Autodesk Fusion 360 part; units mm, degrees
(part 4 of 5)
sketch "Content (4)" plane through (0, 0, 0) normal (0, 0, 1) x (1, 0, 0) in component "Back"
  line L0 (128, -33) -> (128, -39)
  line L1 (116, -39) -> (116, -33)
  circle A0 centre (172, -18) radius 1.75
  circle A1 centre (182, -28) radius 1.75
  circle A2 centre (182, -18) radius 1.75
  line L2 (2, -6) -> (2, -66) construction
  line L3 (119, -30) -> (125, -30)
  line L4 (242, -6) -> (2, -6) construction
  line L5 (2, -66) -> (242, -66) construction
  circle A3 centre (56, -27) radius 1.5
  circle A4 centre (172, -28) radius 1.75
  circle A5 centre (71, -17) radius 1.5
  circle A6 centre (56, -17) radius 1.5
  circle A7 centre (46, -32) radius 1.5
  circle A8 centre (223.2, -48) radius 5.5
  line L6 (242, -66) -> (242, -6) construction
  circle A9 centre (66, -32) radius 1.5
  circle A10 centre (66, -22) radius 1.5
  circle A11 centre (61, -32) radius 1.5
  circle A12 centre (41, -27) radius 1.5
  circle A13 centre (71, -32) radius 1.5
  circle A14 centre (46, -17) radius 1.5
  circle A15 centre (56, -22) radius 1.5
  circle A16 centre (66, -17) radius 1.5
  circle A17 centre (56, -32) radius 1.5
  circle A18 centre (66, -27) radius 1.5
  circle A19 centre (61, -22) radius 1.5
  circle A20 centre (61, -17) radius 1.5
  circle A21 centre (46, -22) radius 1.5
  circle A22 centre (51, -22) radius 1.5
  line L7 (125, -42) -> (119, -42)
  circle A23 centre (41, -32) radius 1.5
  circle A24 centre (51, -32) radius 1.5
  circle A25 centre (41, -17) radius 1.5
  circle A26 centre (71, -27) radius 1.5
  circle A27 centre (46, -27) radius 1.5
  circle A28 centre (51, -27) radius 1.5
  circle A29 centre (61, -27) radius 1.5
  circle A30 centre (51, -17) radius 1.5
  circle A31 centre (41, -22) radius 1.5
  circle A32 centre (71, -22) radius 1.5
  line L8 (0, 1.75) -> (0, 22.5) construction
  line L9 (1.75, 0) -> (22.5, 0) construction
  circle A33 centre (192, -18) radius 1.75
  circle A34 centre (202, -18) radius 1.75
  circle A35 centre (192, -28) radius 1.75
  circle A36 centre (202, -28) radius 1.75
  line L10 (14.1495, -52.3784) -> (48.441, -52.3784) construction
  line L11 (48.441, -52.3784) -> (48.441, -46.5889) construction
  line L12 (48.441, -46.5889) -> (14.1495, -46.5889) construction
  line L13 (14.1495, -46.5889) -> (14.1495, -52.3784) construction
  arc A37 (119, -30) -> (116, -33) centre (119, -33) ccw
  arc A38 (128, -33) -> (125, -30) centre (125, -33) ccw
  arc A39 (125, -42) -> (128, -39) centre (125, -39) ccw
  arc A40 (116, -39) -> (119, -42) centre (119, -39) ccw
  line L14 (227, -16) -> (227, -26)
  line L15 (220.6, -14) -> (225, -14)
  line L16 (225, -28) -> (220.6, -28)
  line L17 (218.6, -26) -> (218.6, -16)
  arc A41 (220.6, -14) -> (218.6, -16) centre (220.6, -16) ccw
  arc A42 (227, -16) -> (225, -14) centre (225, -16) ccw
  arc A43 (218.6, -26) -> (220.6, -28) centre (220.6, -26) ccw
  arc A44 (225, -28) -> (227, -26) centre (225, -26) ccw
  point P0 (242, -36)
  point P1 (116, -42)
  point P2 (116, -30)
  point P3 (128, -30)
  point P4 (218.6, -28)
  point P5 (218.6, -14)
  point P6 (227, -14)
  point P7 (223.2, -28)
  dimension "d1005" = 5
  dimension "d1006" = 5
  dimension "d1009" = 10
  dimension "d1010" = -10
  dimension "d502" = 240
  dimension "d503" = 60
  dimension "d696" = 18
  dimension "d866" = 12
  dimension "d867" = 12
  dimension "d869" = 24
  dimension "d870" = 3
  dimension "d1039" = 34
  dimension "d1041" = 12
  dimension "d1179" = 18.8
  dimension "d1180" = 114
  dimension "d1183" = 39
  dimension "d1047" = 2
  dimension "d1048" = 6
  dimension "d1561" = 3.5
  dimension "d1562" = 11
  dimension "d1563" = 70
  dimension "d1596" = 3
  dimension "d1597" = 3
  dimension "d1598" = 3
  dimension "d1599" = 3
  dimension "d1646" = 8.4
  dimension "d1647" = 14
  dimension "d1648" = 8
  dimension "d1654" = 2
  dimension "d1655" = 2
  dimension "d1656" = 2
  dimension "d1657" = 2
  dimension "d1658" = 15
  constraint horizontal L5
  constraint vertical L6
  constraint vertical L2
  constraint midpoint P0 L6
  constraint horizontal L4
  constraint horizontal L3
  constraint vertical L0
  constraint horizontal L7
  constraint vertical L1
  constraint coincident P2 L1
  constraint coincident P2 L3
  constraint tangent L1 A37
  constraint tangent L3 A37
  constraint coincident P3 L3
  constraint coincident P3 L0
  constraint tangent L3 A38
  constraint tangent L0 A38
  constraint tangent L0 A39
  constraint tangent L7 A39
  constraint coincident P1 L1
  constraint coincident P1 L7
  constraint tangent L1 A40
  constraint tangent L7 A40
  constraint horizontal L15
  constraint vertical L14
  constraint horizontal L16
  constraint vertical L17
  constraint vertical A8.centre P7
  constraint coincident P5 L17
  constraint coincident P5 L15
  constraint tangent L17 A41
  constraint tangent L15 A41
  constraint coincident P6 L15
  constraint coincident P6 L14
  constraint tangent L15 A42
  constraint tangent L14 A42
  constraint coincident L16 P7
  constraint coincident P4 L17
  constraint coincident P4 L16
  constraint tangent L17 A43
  constraint tangent L16 A43
  constraint tangent L14 A44
  constraint tangent L16 A44
  measures "d502" distance of L5.end L2.end
  measures "d503" distance of L2.end L2.start
  measures "d696" distance of A8.centre L5
  measures "d866" distance of P2 P3
  measures "d867" distance of P1 P2
  measures "d869" distance of L5 L7
  measures "d870" diameter of A23
  measures "d1039" distance of A23.centre L5
  measures "d1041" distance of A0.centre L4
  measures "d1179" distance of A8.centre L6
  measures "d1180" distance of L0 L6
  measures "d1183" distance of A23.centre L2
  measures "d1047" distance of L2 L8
  measures "d1048" distance of L4 L9
  measures "d1561" diameter of A0
  measures "d1562" diameter of A8
  measures "d1563" distance of A0.centre L6
  measures "d1596" radius of A37
  measures "d1597" radius of A38
  measures "d1598" radius of A39
  measures "d1599" radius of A40
  measures "d1646" distance of P5 P6
  measures "d1647" distance of P4 P5
  measures "d1648" distance of L4 L15
  measures "d1654" radius of A41
  measures "d1655" radius of A42
  measures "d1656" radius of A43
  measures "d1657" radius of A44
  measures "d1658" distance of L6 L14
sketch "Content (5)" plane through (0, 0, 0) normal (0, 0, 1) x (1, 0, 0) in component "Right"
  line L0 (-302, 182) -> (-242, 182) construction
  circle A0 centre (-275, 112) radius 5.75
  circle A1 centre (-277, 80) radius 1.75
  circle A2 centre (-287, 100) radius 1.75
  circle A3 centre (-277, 90) radius 1.75
  line L1 (-264.7, 57.5) -> (-267, 57.5)
  line L2 (-267, 45) -> (-264.7, 45)
  circle A4 centre (-287, 90) radius 1.75
  circle A5 centre (-287, 80) radius 1.75
  line L3 (-269, 55.5) -> (-269, 47)
  line L4 (-262.7, 47) -> (-262.7, 55.5)
  circle A6 centre (-297, 151) radius 1
  circle A7 centre (-277, 100) radius 1.75
  circle A8 centre (-297, 61) radius 1
  circle A9 centre (-297, 121) radius 1
  circle A10 centre (-297, 91) radius 1
  line L5 (-242, 182) -> (-242, 0) construction
  circle A11 centre (-297, 31) radius 1
  line L6 (-302, 0) -> (-302, 182) construction
  circle A12 centre (-267, 80) radius 1.75
  line L7 (-242, 0) -> (-302, 0) construction
  circle A13 centre (-267, 90) radius 1.75
  circle A14 centre (-267, 100) radius 1.75
  line L8 (1.75, 0) -> (22.5, 0) construction
  line L9 (0, 1.75) -> (0, 22.5) construction
  arc A15 (-262.7, 55.5) -> (-264.7, 57.5) centre (-264.7, 55.5) ccw
  arc A16 (-267, 57.5) -> (-269, 55.5) centre (-267, 55.5) ccw
  arc A17 (-269, 47) -> (-267, 45) centre (-267, 47) ccw
  arc A18 (-264.7, 45) -> (-262.7, 47) centre (-264.7, 47) ccw
  point P0 (-242, 91)
  point P1 (-262.7, 45)
  point P2 (-272, 0)
  point P3 (-269, 45)
  point P4 (-269, 57.5)
  point P5 (-302, 182)
  point P6 (-272, 182)
  dimension "d960" = -10
  dimension "d961" = -10
  dimension "d964" = 0
  dimension "d965" = -30
  dimension "d846" = 2
  dimension "d910" = 182
  dimension "d911" = 60
  dimension "d923" = 11.5
  dimension "d924" = 70
  dimension "d925" = 27
  dimension "d927" = 33
  dimension "d929" = 6.3
  dimension "d930" = 3.5
  dimension "d1192" = 100
  dimension "d1194" = 91
  dimension "d992" = 12.5
  dimension "d993" = 242
  dimension "d1538" = 45
  dimension "d1540" = 15
  dimension "d1564" = 5
  dimension "d1642" = 2
  dimension "d1643" = 2
  dimension "d1644" = 2
  dimension "d1645" = 2
  constraint perpendicular L5 L7
  constraint parallel L5 L6
  constraint coincident P5 L0.start
  constraint perpendicular L0 L5
  constraint midpoint P2 L7
  constraint midpoint P6 L0
  constraint horizontal L2
  constraint horizontal L1
  constraint vertical L3
  constraint midpoint P0 L5
  constraint perpendicular L1 L4
  constraint collinear L7 L8
  constraint tangent L1 A15
  constraint tangent L4 A15
  constraint coincident P4 L1
  constraint coincident P4 L3
  constraint tangent L1 A16
  constraint tangent L3 A16
  constraint coincident P3 L3
  constraint coincident P3 L2
  constraint tangent L3 A17
  constraint tangent L2 A17
  constraint coincident P1 L2
  constraint coincident P1 L4
  constraint tangent L2 A18
  constraint tangent L4 A18
  measures "d846" diameter of A10
  measures "d910" distance of L6.start P5
  measures "d911" distance of L6.start L5.end
  measures "d923" diameter of A0
  measures "d924" distance of A0.centre L0
  measures "d925" distance of A0.centre L6
  measures "d927" distance of L3 L6
  measures "d929" distance of P1 P3
  measures "d930" diameter of A14
  measures "d1192" distance of A14.centre L7
  measures "d1194" distance of A10.centre L7
  measures "d992" distance of P3 P4
  measures "d993" distance of L5 L9
  measures "d1538" distance of L2 L7
  measures "d1540" distance of A2.centre L6
  measures "d1564" distance of A10.centre L6
  measures "d1642" radius of A15
  measures "d1643" radius of A16
  measures "d1644" radius of A17
  measures "d1645" radius of A18
sketch "Content (6)" plane through (0, 0, 0) normal (0, 0, 1) x (1, 0, 0) in component "Left"
  circle A0 centre (-246.401, -121.7005) radius 1
  line L0 (-242, 0) -> (-242, -183.401)
  line L1 (-302, -183.401) -> (-302, -1.401)
  circle A1 centre (-246.401, -31.7005) radius 1
  circle A2 centre (-246.401, -151.7005) radius 1
  circle A3 centre (-246.401, -61.7005) radius 1
  circle A4 centre (-247, -91.7005) radius 1
  line L2 (0, 1.75) -> (0, 22.5) construction
  line L3 (-302, -1.401) -> (-242, -1.401)
  line L4 (-242, -183.401) -> (-302, -183.401)
  line L5 (1.75, 0) -> (22.5, 0) construction
  line L6 (-242, 0) -> (-302, 0)
  circle A5 centre (-247.5, -159.401) radius 1.5
  circle A6 centre (-272, -159.401) radius 20.5 construction
  circle A7 centre (-272, -159.401) radius 15
  circle A8 centre (-296.5, -159.401) radius 1.5
  line L7 (-296.5, -159.401) -> (-247.5, -159.401) construction
  circle A9 centre (-272, -113.401) radius 20.5 construction
  circle A10 centre (-296.5, -113.401) radius 1.5
  line L8 (-296.5, -113.401) -> (-247.5, -113.401) construction
  circle A11 centre (-272, -113.401) radius 15
  circle A12 centre (-272, -67.401) radius 20.5 construction
  circle A13 centre (-296.5, -67.401) radius 1.5
  line L9 (-296.5, -67.401) -> (-247.5, -67.401) construction
  circle A14 centre (-272, -67.401) radius 15
  circle A15 centre (-247.5, -113.401) radius 1.5
  circle A16 centre (-247.5, -67.401) radius 1.5
  circle A17 centre (-262.9095, -67.5364) radius 3.5
  circle A18 centre (-262.9095, -67.5364) radius 1.6
  circle A19 centre (-267.3375, -59.5961) radius 1.6
  circle A20 centre (-267.3375, -59.5961) radius 3.5
  circle A21 centre (-276.428, -59.4607) radius 1.6
  circle A22 centre (-276.428, -59.4607) radius 3.5
  circle A23 centre (-281.0905, -67.2656) radius 1.6
  circle A24 centre (-281.0905, -67.2656) radius 3.5
  circle A25 centre (-276.6625, -75.2059) radius 1.6
  circle A26 centre (-276.6625, -75.2059) radius 3.5
  circle A27 centre (-267.572, -75.3413) radius 1.6
  circle A28 centre (-267.572, -75.3413) radius 3.5
  arc A29 (-267.7994, -108.87) -> (-270.4355, -115.6711) centre (-260.4356, -115.6357) ccw
  line L10 (-270.4355, -115.6711) -> (-270.3981, -126.2293)
  line L11 (-272.3981, -126.2293) -> (-272.4354, -115.699)
  line L12 (-270.3981, -126.2293) -> (-272.4073, -102.4695) construction
  arc A30 (-267.7994, -108.87) -> (-275.1326, -108.9029) centre (-271.4813, -105.4871) ccw
  arc A31 (-272.4354, -115.699) -> (-275.1326, -108.9029) centre (-282.4354, -115.7344) ccw
  line L13 (-272.3981, -126.2293) -> (-270.6073, -102.4695) construction
  line L14 (-272.3981, -126.2293) -> (-270.3981, -126.2293)
  arc A32 (-267.7994, -155.07) -> (-275.1326, -155.1029) centre (-271.4813, -151.6871) ccw
  arc A33 (-267.7994, -155.07) -> (-270.4355, -161.8711) centre (-260.4356, -161.8357) ccw
  line L15 (-272.3981, -172.4293) -> (-272.4354, -161.899)
  line L16 (-270.4355, -161.8711) -> (-270.3981, -172.4293)
  line L17 (-295.901, -159.601) -> (-246.901, -159.601) construction
  arc A34 (-272.4354, -161.899) -> (-275.1326, -155.1029) centre (-282.4354, -161.9344) ccw
  line L18 (-272.3981, -172.4293) -> (-270.6073, -148.6695) construction
  line L19 (-270.3981, -172.4293) -> (-272.4073, -148.6695) construction
  line L20 (-272.3981, -172.4293) -> (-270.3981, -172.4293)
  point P0 (-241.401, -91.7005)
  point P1 (-301.401, -92.401)
  point P2 (-302, -1.401)
  point P3 (-278.401, 0)
  point P4 (-272, -183.401)
  point P5 (-271.4556, -113.7241)
  point P6 (-271.4556, -159.9241)
  point P7 (-271.401, -159.601)
  point P8 (-271.401, -159.601)
  dimension "d523" = 182
  dimension "d861" = 5
  dimension "d1401" = 242
  dimension "d1542" = 60
  dimension "d1763" = 30
  dimension "d1765" = 41
  dimension "d1766" = 3
  dimension "d1767" = 24.5
  dimension "d1768" = 24.5
  dimension "d1769" = 24
  dimension "d1772" = 0
  dimension "d1773" = 46
  dimension "d1778" = 3.2
  dimension "d1779" = 7
  dimension "d1783" = 360
  dimension "d1788" = 1.8
  dimension "d1789" = 10
  dimension "d1790" = 10
  dimension "d1791" = 10
  dimension "d1792" = 1.8
  dimension "d1793" = 10
  dimension "d1794" = 10
  dimension "d1795" = 10
  constraint parallel L0 L1
  constraint coincident P2 L1.end
  constraint horizontal L4
  constraint coincident L1.start L4.end
  constraint coincident L0.start L6.start
  constraint concentric A6 A7
  constraint coincident A8.centre L7.start
  constraint coincident A5.centre L7.end
  constraint coincident A6.centre L7
  constraint equal A5 A8
  constraint horizontal L7
  constraint midpoint L4 P4
  constraint vertical A6.centre P4
  constraint concentric A17 A18
  constraint parallel L10 L11
  constraint coincident P5 L12
  constraint coincident P5 L13
  constraint tangent A29 A30
  constraint tangent A29 L10
  constraint tangent A30 A31
  constraint tangent L11 A31
  constraint horizontal L14
  constraint parallel L15 L16
  constraint coincident P6 L19
  constraint coincident P6 L18
  constraint tangent A32 A33
  constraint tangent A33 L16
  constraint tangent A32 A34
  constraint tangent L15 A34
  constraint horizontal L20
  measures "d523" distance of P2 L1.start
  measures "d861" distance of A4.centre L0
  measures "d1401" distance of L0 L2
  measures "d1542" distance of L0.end L1.start
  measures "d1763" diameter of A7
  measures "d1765" diameter of A6
  measures "d1766" diameter of A5
  measures "d1767" distance of A8.centre A6.centre
  measures "d1768" distance of A5.centre A6.centre
  measures "d1769" distance of L4 A6.centre
  measures "d1778" diameter of A18
  measures "d1779" diameter of A17
  measures "d1788" distance of L12.end L13.end
  measures "d1789" diameter of A30
  measures "d1790" radius of A29
  measures "d1791" radius of A31
  measures "d1792" distance of L19.end L18.end
  measures "d1793" diameter of A32
  measures "d1794" radius of A33
  measures "d1795" radius of A34
sketch "Teeth" plane through (0, 0, 0) normal (0, 0, 1) x (1, 0, 0) in component "Front"
  line L0 (86, 6.3042) -> (86, 15.7758)
  line L1 (89.175, 6.3042) -> (89.175, 15.7758)
  line L2 (87.6137, 36.905) -> (87.5613, 36.905)
  line L3 (87.5613, 27.095) -> (87.6137, 27.095)
  line L4 (87.6137, 16.905) -> (87.5613, 16.905)
  line L5 (89.175, 35.7758) -> (89.175, 28.2242)
  line L6 (89.175, 48.2242) -> (89.175, 57.6958)
  line L7 (86, 57.6958) -> (86, 48.2242)
  line L8 (242, 62) -> (242, 2) construction
  line L9 (2, 2) -> (242, 2) construction
  line L10 (2, 62) -> (2, 2) construction
  arc A0 (87.6137, 16.905) -> (86, 15.7758) centre (86.7071, 16.4829) ccw
  arc A1 (89.175, 15.7758) -> (87.5613, 16.905) centre (88.4679, 16.4829) ccw
  arc A2 (87.5613, 27.095) -> (89.175, 28.2242) centre (88.4679, 27.5171) ccw
  arc A3 (86, 28.2242) -> (87.6137, 27.095) centre (86.7071, 27.5171) ccw
  line L11 (86, 28.2242) -> (86, 35.7758)
  arc A4 (89.175, 35.7758) -> (87.5613, 36.905) centre (88.4679, 36.4829) ccw
  arc A5 (87.6137, 36.905) -> (86, 35.7758) centre (86.7071, 36.4829) ccw
  arc A6 (87.5613, 47.095) -> (89.175, 48.2242) centre (88.4679, 47.5171) ccw
  arc A7 (86, 48.2242) -> (87.6137, 47.095) centre (86.7071, 47.5171) ccw
  line L12 (0, 1.75) -> (0, 22.5) construction
  line L13 (87.5613, 47.095) -> (87.6137, 47.095)
  line L14 (87.6137, 58.825) -> (87.5613, 58.825)
  line L15 (2, 62) -> (242, 62) construction
  line L16 (1.75, 0) -> (22.5, 0)
  line L17 (87.6137, 5.175) -> (87.5613, 5.175)
  arc A8 (87.6137, 58.825) -> (86, 57.6958) centre (86.7071, 58.4029) ccw
  arc A9 (89.175, 57.6958) -> (87.5613, 58.825) centre (88.4679, 58.4029) ccw
  arc A10 (86, 6.3042) -> (87.6137, 5.175) centre (86.7071, 5.5971) ccw
  arc A11 (87.5613, 5.175) -> (89.175, 6.3042) centre (88.4679, 5.5971) ccw
  dimension "d1086" = 2
  dimension "d1087" = 0.4221
  dimension "d1091" = 10.19
  dimension "d1094" = 2
  dimension "d1109" = 0.4221
  dimension "d1113" = 2
  dimension "d1116" = 3.175
  dimension "d1117" = 0.7071
  dimension "d1221" = 2
  dimension "d1222" = 2
  dimension "d1223" = 2
  dimension "d1224" = 2
  dimension "d1225" = 2
  dimension "d1227" = 0.7071
  dimension "d1228" = 0.7071
  dimension "d1229" = 0.4221
  dimension "d1230" = 0.4221
  dimension "d1232" = 0.4221
  dimension "d1233" = 0.4221
  dimension "d1235" = 0.7071
  dimension "d1236" = 0.7071
  dimension "d1178" = 0.7071
  dimension "d1323" = 240
  dimension "d1324" = 84
  dimension "d1399" = 2
  dimension "d1454" = 3.175
  dimension "d1456" = 0.4221
  dimension "d1457" = 0.4221
  dimension "d1460" = 60
  dimension "d1461" = 2
  dimension "d1462" = 3.175
  dimension "d1463" = 3.175
  dimension "d1466" = 9.81
  dimension "d1468" = 14.905
  dimension "d1469" = 14.905
  dimension "d1471" = 10.19
  dimension "d1472" = 0.7071
  dimension "d1473" = 0.7071
  dimension "d1571" = 2
  dimension "d1573" = 2
  dimension "d1574" = 0.7071
  dimension "d1575" = 0.7071
  dimension "d1576" = 0.4221
  dimension "d1577" = 0.4221
  dimension "d1578" = 2
  dimension "d1579" = 2
  dimension "d1580" = 0.4221
  dimension "d1581" = 0.4221
  dimension "d1582" = 0.7071
  dimension "d1583" = 0.7071
  constraint vertical L7
  constraint vertical L6
  constraint horizontal L3
  constraint horizontal L2
  constraint vertical L5
  constraint collinear L1 L5
  constraint perpendicular L9 L10
  constraint collinear L0 L11
  constraint collinear L7 L11
  constraint horizontal L13
  constraint perpendicular L7 L14
  constraint perpendicular L8 L15
  constraint perpendicular L0 L17
  measures "d1086" diameter of A0
  measures "d1087" distance of A0.centre L4
  measures "d1091" distance of L3 L4
  measures "d1094" diameter of A7
  measures "d1109" distance of A5.centre L2
  measures "d1113" diameter of A5
  measures "d1116" distance of L6 L7
  measures "d1117" distance of A7.centre L7
  measures "d1221" diameter of A1
  measures "d1222" diameter of A2
  measures "d1223" diameter of A4
  measures "d1224" diameter of A3
  measures "d1225" diameter of A6
  measures "d1227" distance of A6.centre L6
  measures "d1228" distance of A0.centre L0
  measures "d1229" distance of A1.centre L4
  measures "d1230" distance of A2.centre L3
  measures "d1232" distance of A3.centre L3
  measures "d1233" distance of A4.centre L2
  measures "d1235" distance of A4.centre L5
  measures "d1236" distance of A2.centre L5
  measures "d1178" distance of A1.centre L1
  measures "d1323" distance of L10.start L8.start
  measures "d1324" distance of L0 L10
  measures "d1399" distance of L10 L12
  measures "d1454" distance of L5 L11
  measures "d1456" distance of A6.centre L13
  measures "d1457" distance of A7.centre L13
  measures "d1460" distance of L9 L15
  measures "d1461" distance of L9 L16
  measures "d1462" distance of L14 L15
  measures "d1463" distance of L9 L17
  measures "d1466" distance of L2 L3
  measures "d1468" distance of L4 L9
  measures "d1469" distance of L13 L15
  measures "d1471" distance of L2 L13
  measures "d1472" distance of A3.centre L11
  measures "d1473" distance of A5.centre L11
  measures "d1571" diameter of A10
  measures "d1573" diameter of A11
  measures "d1574" distance of L0 A10.centre
  measures "d1575" distance of L1 A11.centre
  measures "d1576" distance of L17 A11.centre
  measures "d1577" distance of L17 A10.centre
  measures "d1578" diameter of A8
  measures "d1579" diameter of A9
  measures "d1580" distance of L14 A8.centre
  measures "d1581" distance of L14 A9.centre
  measures "d1582" distance of L7 A8.centre
  measures "d1583" distance of L6 A9.centre
sketch "Teeth (2)" plane through (0, 0, 0) normal (0, 0, 1) x (1, 0, 0) in component "Back"
  arc A0 (86, -39.7758) -> (87.6137, -40.905) centre (86.7071, -40.4829) ccw
  arc A1 (89.175, -52.2242) -> (87.5613, -51.095) centre (88.4679, -51.5171) ccw
  line L0 (2, -6) -> (2, -66) construction
  line L1 (87.6137, -31.095) -> (87.5613, -31.095)
  line L2 (89.175, -32.2242) -> (89.175, -39.7758)
  line L3 (89.175, -61.6958) -> (89.175, -52.2242)
  line L4 (87.5613, -20.905) -> (87.6137, -20.905)
  line L5 (86, -10.3042) -> (86, -19.7758)
  arc A2 (89.175, -32.2242) -> (87.5613, -31.095) centre (88.4679, -31.5171) ccw
  arc A3 (87.6137, -31.095) -> (86, -32.2242) centre (86.7071, -31.5171) ccw
  arc A4 (87.5613, -20.905) -> (89.175, -19.7758) centre (88.4679, -20.4829) ccw
  arc A5 (86, -19.7758) -> (87.6137, -20.905) centre (86.7071, -20.4829) ccw
  line L6 (87.5613, -40.905) -> (87.6137, -40.905)
  line L7 (89.175, -19.7758) -> (89.175, -10.3042)
  line L8 (86, -61.6958) -> (86, -52.2242)
  line L9 (87.6137, -51.095) -> (87.5613, -51.095)
  arc A6 (87.6137, -51.095) -> (86, -52.2242) centre (86.7071, -51.5171) ccw
  arc A7 (87.5613, -40.905) -> (89.175, -39.7758) centre (88.4679, -40.4829) ccw
  line L10 (2, -6) -> (80.576, -6) construction
  line L11 (242, -6) -> (242, -66) construction
  line L12 (0, 1.75) -> (0, 22.5) construction
  line L13 (1.75, 0) -> (22.5, 0) construction
  line L14 (86, -32.2242) -> (86, -39.7758)
  line L15 (77.401, -66) -> (242, -66) construction
  line L16 (2, -66) -> (77.401, -66) construction
  line L17 (87.6137, -62.825) -> (87.5613, -62.825)
  line L18 (80.576, -6) -> (242, -6) construction
  line L19 (87.6137, -9.175) -> (87.5613, -9.175)
  arc A8 (87.5613, -62.825) -> (89.175, -61.6958) centre (88.4679, -62.4029) ccw
  arc A9 (86, -61.6958) -> (87.6137, -62.825) centre (86.7071, -62.4029) ccw
  arc A10 (87.6137, -9.175) -> (86, -10.3042) centre (86.7071, -9.5971) ccw
  arc A11 (89.175, -10.3042) -> (87.5613, -9.175) centre (88.4679, -9.5971) ccw
  dimension "d1404" = 2
  dimension "d1405" = 0.4221
  dimension "d1406" = 10.19
  dimension "d1407" = 2
  dimension "d1408" = 0.4221
  dimension "d1409" = 2
  dimension "d1412" = 0.7071
  dimension "d1413" = 2
  dimension "d1414" = 2
  dimension "d1415" = 2
  dimension "d1416" = 2
  dimension "d1417" = 2
  dimension "d1418" = 0.7071
  dimension "d1419" = 0.7071
  dimension "d1420" = 0.4221
  dimension "d1421" = 0.4221
  dimension "d1423" = 0.4221
  dimension "d1424" = 0.4221
  dimension "d1425" = 0.7071
  dimension "d1426" = 0.7071
  dimension "d1427" = 0.7071
  dimension "d1428" = 240
  dimension "d1429" = 84
  dimension "d1431" = 14.905
  dimension "d1433" = 9.81
  dimension "d1436" = 2
  dimension "d1437" = 14.905
  dimension "d1440" = 6
  dimension "d1441" = 0.4221
  dimension "d1442" = 0.4221
  dimension "d1443" = 0.7071
  dimension "d1444" = 0.7071
  dimension "d1446" = 3.175
  dimension "d1447" = 3.175
  dimension "d1451" = 3.175
  dimension "d1452" = 60
  dimension "d1453" = 3.175
  dimension "d1470" = 10.19
  dimension "d1584" = 2
  dimension "d1585" = 2
  dimension "d1586" = 0.7071
  dimension "d1587" = 0.4221
  dimension "d1588" = 0.4221
  dimension "d1589" = 0.7071
  dimension "d1590" = 2
  dimension "d1591" = 2
  dimension "d1592" = 0.7071
  dimension "d1593" = 0.7071
  dimension "d1594" = 0.4221
  dimension "d1595" = 0.4221
  constraint vertical L5
  constraint vertical L7
  constraint horizontal L6
  constraint horizontal L1
  constraint vertical L2
  constraint collinear L2 L3
  constraint perpendicular L0 L10
  constraint perpendicular L0 L16
  constraint collinear L8 L14
  constraint perpendicular L8 L17
  constraint collinear L5 L14
  constraint perpendicular L5 L19
  measures "d1404" diameter of A6
  measures "d1405" distance of A6.centre L9
  measures "d1406" distance of L6 L9
  measures "d1407" diameter of A5
  measures "d1408" distance of A3.centre L1
  measures "d1409" diameter of A3
  measures "d1412" distance of A5.centre L5
  measures "d1413" diameter of A1
  measures "d1414" diameter of A7
  measures "d1415" diameter of A2
  measures "d1416" diameter of A0
  measures "d1417" diameter of A4
  measures "d1418" distance of A4.centre L7
  measures "d1419" distance of A6.centre L8
  measures "d1420" distance of A1.centre L9
  measures "d1421" distance of A7.centre L6
  measures "d1423" distance of A0.centre L6
  measures "d1424" distance of A2.centre L1
  measures "d1425" distance of A2.centre L2
  measures "d1426" distance of A7.centre L2
  measures "d1427" distance of A1.centre L3
  measures "d1428" distance of L0.start L11.start
  measures "d1429" distance of L0 L8
  measures "d1431" distance of L9 L15
  measures "d1433" distance of L1 L6
  measures "d1436" distance of L0 L12
  measures "d1437" distance of L4 L10
  measures "d1440" distance of L10 L13
  measures "d1441" distance of A5.centre L4
  measures "d1442" distance of A4.centre L4
  measures "d1443" horizontal distance of A3.centre A3.end
  measures "d1444" distance of A0.centre L14
  measures "d1446" distance of L5 L7
  measures "d1447" distance of L2 L14
  measures "d1451" distance of L16 L17
  measures "d1452" distance of L10 L15
  measures "d1453" distance of L10 L19
  measures "d1470" distance of L1 L4
  measures "d1584" diameter of A9
  measures "d1585" diameter of A8
  measures "d1586" distance of L8 A9.centre
  measures "d1587" distance of L17 A9.centre
  measures "d1588" distance of L17 A8.centre
  measures "d1589" distance of L3 A8.centre
  measures "d1590" diameter of A10
  measures "d1591" diameter of A11
  measures "d1592" distance of L5 A10.centre
  measures "d1593" distance of L7 A11.centre
  measures "d1594" distance of L19 A10.centre
  measures "d1595" distance of L19 A11.centre
sketch "Fingers Bottom" plane through (0, 0, 0) normal (0, 0, 1) x (1, 0, 0) in component "Bottom"
  arc A0 (-85.6137, -27.905) -> (-84, -26.7758) centre (-84.7071, -27.4829) ccw
  arc A1 (-84, -119.2242) -> (-85.6137, -118.095) centre (-84.7071, -118.5171) ccw
  arc A2 (-84, -39.2242) -> (-85.6137, -38.095) centre (-84.7071, -38.5171) ccw
  line L0 (-84, -26.7758) -> (-84, -19.2242)
  arc A3 (-85.6137, -107.905) -> (-84, -106.7758) centre (-84.7071, -107.4829) ccw
  arc A4 (-87.175, -126.7758) -> (-85.5613, -127.905) centre (-86.4679, -127.4829) ccw
  arc A5 (-84, -139.2242) -> (-85.6137, -138.095) centre (-84.7071, -138.5171) ccw
  line L1 (-84, -146.7758) -> (-84, -139.2242)
  line L2 (-85.5613, -107.905) -> (-85.6137, -107.905)
  arc A6 (-87.175, -146.7758) -> (-85.5613, -147.905) centre (-86.4679, -147.4829) ccw
  line L3 (-85.5613, -147.905) -> (-85.6137, -147.905)
  arc A7 (-87.175, -26.7758) -> (-85.5613, -27.905) centre (-86.4679, -27.4829) ccw
  line L4 (-87.175, -119.2242) -> (-87.175, -126.7758)
  line L5 (-85.5613, -127.905) -> (-85.6137, -127.905)
  arc A8 (-85.5613, -18.095) -> (-87.175, -19.2242) centre (-86.4679, -18.5171) ccw
  line L6 (-85.6137, -38.095) -> (-85.5613, -38.095)
  arc A9 (-87.175, -106.7758) -> (-85.5613, -107.905) centre (-86.4679, -107.4829) ccw
  line L7 (-85.6137, -18.095) -> (-85.5613, -18.095)
  line L8 (-85.5613, -27.905) -> (-85.6137, -27.905)
  arc A10 (-85.6137, -127.905) -> (-84, -126.7758) centre (-84.7071, -127.4829) ccw
  line L9 (-85.6137, -118.095) -> (-85.5613, -118.095)
  line L10 (-84, -46.7758) -> (-84, -39.2242)
  arc A11 (-84, -79.2242) -> (-85.6137, -78.095) centre (-84.7071, -78.5171) ccw
  arc A12 (-84, -59.2242) -> (-85.6137, -58.095) centre (-84.7071, -58.5171) ccw
  arc A13 (-85.5613, -58.095) -> (-87.175, -59.2242) centre (-86.4679, -58.5171) ccw
  arc A14 (-87.175, -86.7758) -> (-85.5613, -87.905) centre (-86.4679, -87.4829) ccw
  line L11 (-87.175, -59.2242) -> (-87.175, -66.7758)
  line L12 (0, 0) -> (-240, 0) construction
  line L13 (-85.5613, -47.905) -> (-85.6137, -47.905)
  arc A15 (-87.175, -66.7758) -> (-85.5613, -67.905) centre (-86.4679, -67.4829) ccw
  arc A16 (-87.175, -46.7758) -> (-85.5613, -47.905) centre (-86.4679, -47.4829) ccw
  line L14 (-85.6137, -78.095) -> (-85.5613, -78.095)
  line L15 (-84, -66.7758) -> (-84, -59.2242)
  arc A17 (-85.6137, -47.905) -> (-84, -46.7758) centre (-84.7071, -47.4829) ccw
  line L16 (-87.175, -139.2242) -> (-87.175, -146.7758)
  line L17 (-85.6137, -138.095) -> (-85.5613, -138.095)
  line L18 (-84, -126.7758) -> (-84, -119.2242)
  line L19 (-87.175, -39.2242) -> (-87.175, -46.7758)
  line L20 (-85.6137, -58.095) -> (-85.5613, -58.095)
  arc A18 (-85.6137, -147.905) -> (-84, -146.7758) centre (-84.7071, -147.4829) ccw
  arc A19 (-85.5613, -118.095) -> (-87.175, -119.2242) centre (-86.4679, -118.5171) ccw
  arc A20 (-85.5613, -78.095) -> (-87.175, -79.2242) centre (-86.4679, -78.5171) ccw
  line L21 (-87.175, -99.2242) -> (-87.175, -106.7758)
  arc A21 (-85.5613, -138.095) -> (-87.175, -139.2242) centre (-86.4679, -138.5171) ccw
  line L22 (-87.175, -79.2242) -> (-87.175, -86.7758)
  arc A22 (-84, -99.2242) -> (-85.6137, -98.095) centre (-84.7071, -98.5171) ccw
  line L23 (0, 0) -> (0, -184) construction
  arc A23 (-85.5613, -98.095) -> (-87.175, -99.2242) centre (-86.4679, -98.5171) ccw
  line L24 (-84, -86.7758) -> (-84, -79.2242)
  line L25 (-85.6137, -98.095) -> (-85.5613, -98.095)
  line L26 (-85.5613, -87.905) -> (-85.6137, -87.905)
  arc A24 (-85.6137, -87.905) -> (-84, -86.7758) centre (-84.7071, -87.4829) ccw
  line L27 (0, -184) -> (-240, -184) construction
  line L28 (-240, 0) -> (-240, -184) construction
  line L29 (-85.5613, -67.905) -> (-85.6137, -67.905)
  arc A25 (-85.6137, -67.905) -> (-84, -66.7758) centre (-84.7071, -67.4829) ccw
  arc A26 (-85.5613, -158.095) -> (-87.175, -159.2242) centre (-86.4679, -158.5171) ccw
  arc A27 (-84, -19.2242) -> (-85.6137, -18.095) centre (-84.7071, -18.5171) ccw
  line L30 (-87.175, -19.2242) -> (-87.175, -26.7758)
  arc A28 (-85.6137, -167.905) -> (-84, -166.7758) centre (-84.7071, -167.4829) ccw
  line L31 (-85.6137, -158.095) -> (-85.5613, -158.095)
  line L32 (-84, -166.7758) -> (-84, -159.2242)
  arc A29 (-87.175, -166.7758) -> (-85.5613, -167.905) centre (-86.4679, -167.4829) ccw
  arc A30 (-85.5613, -38.095) -> (-87.175, -39.2242) centre (-86.4679, -38.5171) ccw
  line L33 (-85.5613, -167.905) -> (-85.6137, -167.905)
  line L34 (-87.175, -159.2242) -> (-87.175, -166.7758)
  arc A31 (-84, -159.2242) -> (-85.6137, -158.095) centre (-84.7071, -158.5171) ccw
  line L35 (-84, -106.7758) -> (-84, -99.2242)
  line L36 (-240, -2) -> (0, -2)
  point P0 (0, -184)
  dimension "d1377" = 20
  dimension "d1378" = 20
  dimension "d1379" = 2
  dimension "d1380" = 0.4221
  dimension "d1381" = 9.81
  dimension "d1382" = 2
  dimension "d1383" = 16.095
  dimension "d1384" = 3.175
  dimension "d1385" = 2
  dimension "d1386" = 2
  dimension "d1387" = 0.4221
  dimension "d1388" = 0.4221
  dimension "d1389" = 0.7071
  dimension "d1390" = 0.7071
  dimension "d1391" = 0.7071
  dimension "d1392" = 84
  dimension "d1393" = 0.4221
  dimension "d1395" = 240
  dimension "d1622" = 182
  constraint horizontal L27
  constraint perpendicular L32 L33
  constraint vertical A28.centre A31.centre
  constraint perpendicular L12 L23
  constraint perpendicular L27 L28
  constraint coincident P0 L23.end
  constraint coincident L12.start L23.start
  measures "d1379" diameter of A31
  measures "d1380" distance of A31.centre L31
  measures "d1381" distance of L31 L33
  measures "d1382" diameter of A28
  measures "d1383" distance of L27 L33
  measures "d1384" distance of L32 L34
  measures "d1385" diameter of A26
  measures "d1386" diameter of A29
  measures "d1387" distance of A26.centre L31
  measures "d1388" distance of A29.centre L33
  measures "d1389" distance of A29.centre L34
  measures "d1390" distance of A28.centre L32
  measures "d1391" distance of A26.centre L34
  measures "d1392" distance of L23 L32
  measures "d1393" distance of A28.centre L33
  measures "d1395" distance of L27.end P0
  measures "d1622" distance of L27 L36
sketch "Fingers" plane through (0, 0, 0) normal (0, 0, 1) x (1, 0, 0) in component "Top"
  arc A0 (-85.6137, 16.095) -> (-84, 17.2242) centre (-84.7071, 16.5171) ccw
  arc A1 (-85.6137, 36.095) -> (-84, 37.2242) centre (-84.7071, 36.5171) ccw
  line L0 (-87.175, 44.7758) -> (-87.175, 37.2242)
  arc A2 (-84, 24.7758) -> (-85.6137, 25.905) centre (-84.7071, 25.4829) ccw
  line L1 (-87.175, 24.7758) -> (-87.175, 17.2242)
  line L2 (-87.175, 64.7758) -> (-87.175, 57.2242)
  line L3 (-85.6137, 125.905) -> (-85.5613, 125.905)
  arc A3 (-84, 144.7758) -> (-85.6137, 145.905) centre (-84.7071, 145.4829) ccw
  arc A4 (-85.6137, 156.095) -> (-84, 157.2242) centre (-84.7071, 156.5171) ccw
  arc A5 (-85.5613, 125.905) -> (-87.175, 124.7758) centre (-86.4679, 125.4829) ccw
  line L4 (-87.175, 144.7758) -> (-87.175, 137.2242)
  line L5 (-87.175, 164.7758) -> (-87.175, 157.2242)
  line L6 (-87.175, 104.7758) -> (-87.175, 97.2242)
  line L7 (-85.6137, 145.905) -> (-85.5613, 145.905)
  arc A6 (-85.5613, 105.905) -> (-87.175, 104.7758) centre (-86.4679, 105.4829) ccw
  line L8 (-85.5613, 96.095) -> (-85.6137, 96.095)
  arc A7 (-84, 124.7758) -> (-85.6137, 125.905) centre (-84.7071, 125.4829) ccw
  arc A8 (-87.175, 137.2242) -> (-85.5613, 136.095) centre (-86.4679, 136.5171) ccw
  line L9 (-85.5613, 116.095) -> (-85.6137, 116.095)
  arc A9 (-84, 84.7758) -> (-85.6137, 85.905) centre (-84.7071, 85.4829) ccw
  line L10 (-84, 157.2242) -> (-84, 164.7758)
  line L11 (-85.5613, 156.095) -> (-85.6137, 156.095)
  line L12 (-84, 137.2242) -> (-84, 144.7758)
  arc A10 (-85.6137, 116.095) -> (-84, 117.2242) centre (-84.7071, 116.5171) ccw
  line L13 (-85.6137, 165.905) -> (-85.5613, 165.905)
  arc A11 (-84, 164.7758) -> (-85.6137, 165.905) centre (-84.7071, 165.4829) ccw
  arc A12 (-87.175, 157.2242) -> (-85.5613, 156.095) centre (-86.4679, 156.5171) ccw
  arc A13 (-85.5613, 165.905) -> (-87.175, 164.7758) centre (-86.4679, 165.4829) ccw
  line L14 (-85.6137, 85.905) -> (-85.5613, 85.905)
  arc A14 (-87.175, 117.2242) -> (-85.5613, 116.095) centre (-86.4679, 116.5171) ccw
  arc A15 (-85.6137, 96.095) -> (-84, 97.2242) centre (-84.7071, 96.5171) ccw
  arc A16 (-85.5613, 145.905) -> (-87.175, 144.7758) centre (-86.4679, 145.4829) ccw
  arc A17 (-85.5613, 85.905) -> (-87.175, 84.7758) centre (-86.4679, 85.4829) ccw
  arc A18 (-87.175, 97.2242) -> (-85.5613, 96.095) centre (-86.4679, 96.5171) ccw
  arc A19 (-87.175, 37.2242) -> (-85.5613, 36.095) centre (-86.4679, 36.5171) ccw
  arc A20 (-84, 44.7758) -> (-85.6137, 45.905) centre (-84.7071, 45.4829) ccw
  line L15 (0, 0) -> (-240, 0) construction
  line L16 (-85.5613, 16.095) -> (-85.6137, 16.095)
  arc A21 (-85.5613, 25.905) -> (-87.175, 24.7758) centre (-86.4679, 25.4829) ccw
  line L17 (-85.6137, 65.905) -> (-85.5613, 65.905)
  line L18 (-84, 37.2242) -> (-84, 44.7758)
  line L19 (-85.6137, 45.905) -> (-85.5613, 45.905)
  arc A22 (-87.175, 17.2242) -> (-85.5613, 16.095) centre (-86.4679, 16.5171) ccw
  arc A23 (-87.175, 57.2242) -> (-85.5613, 56.095) centre (-86.4679, 56.5171) ccw
  line L20 (-85.5613, 36.095) -> (-85.6137, 36.095)
  arc A24 (-84, 64.7758) -> (-85.6137, 65.905) centre (-84.7071, 65.4829) ccw
  line L21 (0, 182) -> (-240, 182) construction
  arc A25 (-85.5613, 45.905) -> (-87.175, 44.7758) centre (-86.4679, 45.4829) ccw
  arc A26 (-85.5613, 65.905) -> (-87.175, 64.7758) centre (-86.4679, 65.4829) ccw
  line L22 (-87.175, 84.7758) -> (-87.175, 77.2242)
  line L23 (-84, 57.2242) -> (-84, 64.7758)
  arc A27 (-85.6137, 136.095) -> (-84, 137.2242) centre (-84.7071, 136.5171) ccw
  line L24 (-84, 17.2242) -> (-84, 24.7758)
  line L25 (-85.6137, 25.905) -> (-85.5613, 25.905)
  arc A28 (-85.6137, 56.095) -> (-84, 57.2242) centre (-84.7071, 56.5171) ccw
  line L26 (-240, 182) -> (-240, 0) construction
  line L27 (0, 182) -> (0, 0) construction
  line L28 (-85.5613, 56.095) -> (-85.6137, 56.095)
  line L29 (-84, 77.2242) -> (-84, 84.7758)
  line L30 (-84, 117.2242) -> (-84, 124.7758)
  arc A29 (-87.175, 77.2242) -> (-85.5613, 76.095) centre (-86.4679, 76.5171) ccw
  line L31 (-85.6137, 105.905) -> (-85.5613, 105.905)
  arc A30 (-84, 104.7758) -> (-85.6137, 105.905) centre (-84.7071, 105.4829) ccw
  line L32 (-84, 97.2242) -> (-84, 104.7758)
  line L33 (-87.175, 124.7758) -> (-87.175, 117.2242)
  line L34 (-85.5613, 76.095) -> (-85.6137, 76.095)
  arc A31 (-85.6137, 76.095) -> (-84, 77.2242) centre (-84.7071, 76.5171) ccw
  line L35 (-85.5613, 136.095) -> (-85.6137, 136.095)
  dimension "d1479" = 20
  dimension "d1480" = 20
  dimension "d1481" = 2
  dimension "d1482" = 0.4221
  dimension "d1483" = 9.81
  dimension "d1484" = 2
  dimension "d1485" = 16.095
  dimension "d1486" = 3.175
  dimension "d1487" = 2
  dimension "d1488" = 2
  dimension "d1489" = 0.4221
  dimension "d1490" = 0.4221
  dimension "d1491" = 0.7071
  dimension "d1492" = 0.7071
  dimension "d1493" = 0.7071
  dimension "d1494" = 84
  dimension "d1495" = 0.4221
  dimension "d1496" = 182
  dimension "d1497" = 240
  constraint horizontal L15
  constraint perpendicular L16 L24
  constraint vertical A2.centre A0.centre
  constraint perpendicular L21 L27
  constraint perpendicular L15 L26
  constraint coincident L15.start L27.end
  measures "d1481" diameter of A2
  measures "d1482" distance of A2.centre L25
  measures "d1483" distance of L16 L25
  measures "d1484" diameter of A0
  measures "d1485" distance of L15 L16
  measures "d1486" distance of L1 L24
  measures "d1487" diameter of A21
  measures "d1488" diameter of A22
  measures "d1489" distance of A21.centre L25
  measures "d1490" distance of A22.centre L16
  measures "d1491" distance of A22.centre L1
  measures "d1492" distance of A0.centre L24
  measures "d1493" distance of A21.centre L1
  measures "d1494" distance of L24 L27
  measures "d1495" distance of A0.centre L16
  measures "d1496" distance of L15.start L21.start
  measures "d1497" distance of L15.end L15.start
sketch "Projection" plane through (0, 0, 0) normal (0, 0, 1) x (1, 0, 0) in component "Brace"
  line L0 (3.175, 14.7758) -> (3.175, 0)
  line L1 (3.175, 0) -> (15.095, 0)
  line L2 (15.095, 0) -> (15.095, 1.5613)
  arc A0 (16.2242, 3.175) -> (15.095, 1.5613) centre (15.5171, 2.4679) ccw
  line L3 (16.2242, 3.175) -> (23.7758, 3.175)
  arc A1 (24.905, 1.5613) -> (23.7758, 3.175) centre (24.4829, 2.4679) ccw
  line L4 (24.905, 1.5613) -> (24.905, 0)
  line L5 (24.905, 0) -> (35.095, 0)
  line L6 (35.095, 0) -> (35.095, 1.5613)
  arc A2 (36.2242, 3.175) -> (35.095, 1.5613) centre (35.5171, 2.4679) ccw
  line L7 (36.2242, 3.175) -> (43.7758, 3.175)
  arc A3 (44.905, 1.5613) -> (43.7758, 3.175) centre (44.4829, 2.4679) ccw
  line L8 (44.905, 1.5613) -> (44.905, 0)
  line L9 (44.905, 0) -> (56.825, 0)
  line L10 (56.825, 0) -> (56.825, 14.7758)
  arc A4 (58.4387, 15.905) -> (56.825, 14.7758) centre (57.5321, 15.4829) ccw
  line L11 (58.4387, 15.905) -> (60, 15.905)
  line L12 (60, 15.905) -> (60, 26.095)
  line L13 (60, 26.095) -> (58.4387, 26.095)
  arc A5 (56.825, 27.2242) -> (58.4387, 26.095) centre (57.5321, 26.5171) ccw
  line L14 (56.825, 27.2242) -> (56.825, 34.7758)
  arc A6 (58.4387, 35.905) -> (56.825, 34.7758) centre (57.5321, 35.4829) ccw
  line L15 (58.4387, 35.905) -> (60, 35.905)
  line L16 (60, 35.905) -> (60, 46.095)
  line L17 (60, 46.095) -> (58.4387, 46.095)
  arc A7 (56.825, 47.2242) -> (58.4387, 46.095) centre (57.5321, 46.5171) ccw
  line L18 (56.825, 47.2242) -> (56.825, 54.7758)
  arc A8 (58.4387, 55.905) -> (56.825, 54.7758) centre (57.5321, 55.4829) ccw
  line L19 (58.4387, 55.905) -> (60, 55.905)
  line L20 (60, 55.905) -> (60, 66.095)
  line L21 (60, 66.095) -> (58.4387, 66.095)
  arc A9 (56.825, 67.2242) -> (58.4387, 66.095) centre (57.5321, 66.5171) ccw
  line L22 (56.825, 67.2242) -> (56.825, 74.7758)
  arc A10 (58.4387, 75.905) -> (56.825, 74.7758) centre (57.5321, 75.4829) ccw
  line L23 (58.4387, 75.905) -> (60, 75.905)
  line L24 (60, 75.905) -> (60, 86.095)
  line L25 (60, 86.095) -> (58.4387, 86.095)
  arc A11 (56.825, 87.2242) -> (58.4387, 86.095) centre (57.5321, 86.5171) ccw
  line L26 (56.825, 87.2242) -> (56.825, 94.7758)
  arc A12 (58.4387, 95.905) -> (56.825, 94.7758) centre (57.5321, 95.4829) ccw
  line L27 (58.4387, 95.905) -> (60, 95.905)
  line L28 (60, 95.905) -> (60, 106.095)
  line L29 (60, 106.095) -> (58.4387, 106.095)
  arc A13 (56.825, 107.2242) -> (58.4387, 106.095) centre (57.5321, 106.5171) ccw
  line L30 (56.825, 107.2242) -> (56.825, 114.7758)
  arc A14 (58.4387, 115.905) -> (56.825, 114.7758) centre (57.5321, 115.4829) ccw
  line L31 (58.4387, 115.905) -> (60, 115.905)
  line L32 (60, 115.905) -> (60, 126.095)
  line L33 (60, 126.095) -> (58.4387, 126.095)
  arc A15 (56.825, 127.2242) -> (58.4387, 126.095) centre (57.5321, 126.5171) ccw
  line L34 (56.825, 127.2242) -> (56.825, 134.7758)
  arc A16 (58.4387, 135.905) -> (56.825, 134.7758) centre (57.5321, 135.4829) ccw
  line L35 (58.4387, 135.905) -> (60, 135.905)
  line L36 (60, 135.905) -> (60, 146.095)
  line L37 (60, 146.095) -> (58.4387, 146.095)
  arc A17 (56.825, 147.2242) -> (58.4387, 146.095) centre (57.5321, 146.5171) ccw
  line L38 (56.825, 147.2242) -> (56.825, 154.7758)
  arc A18 (58.4387, 155.905) -> (56.825, 154.7758) centre (57.5321, 155.4829) ccw
  line L39 (58.4387, 155.905) -> (60, 155.905)
  line L40 (60, 155.905) -> (60, 166.095)
  line L41 (60, 166.095) -> (58.4387, 166.095)
  arc A19 (56.825, 167.2242) -> (58.4387, 166.095) centre (57.5321, 166.5171) ccw
  line L42 (56.825, 167.2242) -> (56.825, 182)
  line L43 (56.825, 182) -> (44.905, 182)
  line L44 (44.905, 182) -> (44.905, 180.4387)
  arc A20 (43.7758, 178.825) -> (44.905, 180.4387) centre (44.4829, 179.5321) ccw
  line L45 (43.7758, 178.825) -> (36.2242, 178.825)
  arc A21 (35.095, 180.4387) -> (36.2242, 178.825) centre (35.5171, 179.5321) ccw
  line L46 (35.095, 180.4387) -> (35.095, 182)
  line L47 (35.095, 182) -> (24.905, 182)
  line L48 (24.905, 182) -> (24.905, 180.4387)
  arc A22 (23.7758, 178.825) -> (24.905, 180.4387) centre (24.4829, 179.5321) ccw
  line L49 (23.7758, 178.825) -> (16.2242, 178.825)
  arc A23 (15.095, 180.4387) -> (16.2242, 178.825) centre (15.5171, 179.5321) ccw
  line L50 (15.095, 180.4387) -> (15.095, 182)
  line L51 (15.095, 182) -> (3.175, 182)
  line L52 (3.175, 182) -> (3.175, 167.2242)
  arc A24 (1.5613, 166.095) -> (3.175, 167.2242) centre (2.4679, 166.5171) ccw
  line L53 (1.5613, 166.095) -> (0, 166.095)
  line L54 (0, 166.095) -> (0, 155.905)
  line L55 (0, 155.905) -> (1.5613, 155.905)
  arc A25 (3.175, 154.7758) -> (1.5613, 155.905) centre (2.4679, 155.4829) ccw
  line L56 (3.175, 154.7758) -> (3.175, 147.2242)
  arc A26 (1.5613, 146.095) -> (3.175, 147.2242) centre (2.4679, 146.5171) ccw
  line L57 (1.5613, 146.095) -> (0, 146.095)
  line L58 (0, 146.095) -> (0, 135.905)
  line L59 (0, 135.905) -> (1.5613, 135.905)
  arc A27 (3.175, 134.7758) -> (1.5613, 135.905) centre (2.4679, 135.4829) ccw
  line L60 (3.175, 134.7758) -> (3.175, 127.2242)
  arc A28 (1.5613, 126.095) -> (3.175, 127.2242) centre (2.4679, 126.5171) ccw
  line L61 (1.5613, 126.095) -> (0, 126.095)
  line L62 (0, 126.095) -> (0, 115.905)
  line L63 (0, 115.905) -> (1.5613, 115.905)
  arc A29 (3.175, 114.7758) -> (1.5613, 115.905) centre (2.4679, 115.4829) ccw
  line L64 (3.175, 114.7758) -> (3.175, 107.2242)
  arc A30 (1.5613, 106.095) -> (3.175, 107.2242) centre (2.4679, 106.5171) ccw
  line L65 (1.5613, 106.095) -> (0, 106.095)
  line L66 (0, 106.095) -> (0, 95.905)
  line L67 (0, 95.905) -> (1.5613, 95.905)
  arc A31 (3.175, 94.7758) -> (1.5613, 95.905) centre (2.4679, 95.4829) ccw
  line L68 (3.175, 94.7758) -> (3.175, 87.2242)
  arc A32 (1.5613, 86.095) -> (3.175, 87.2242) centre (2.4679, 86.5171) ccw
  line L69 (1.5613, 86.095) -> (0, 86.095)
  line L70 (0, 86.095) -> (0, 75.905)
  line L71 (0, 75.905) -> (1.5613, 75.905)
  arc A33 (3.175, 74.7758) -> (1.5613, 75.905) centre (2.4679, 75.4829) ccw
  line L72 (3.175, 74.7758) -> (3.175, 67.2242)
  arc A34 (1.5613, 66.095) -> (3.175, 67.2242) centre (2.4679, 66.5171) ccw
  line L73 (1.5613, 66.095) -> (0, 66.095)
  line L74 (0, 66.095) -> (0, 55.905)
  line L75 (0, 55.905) -> (1.5613, 55.905)
  arc A35 (3.175, 54.7758) -> (1.5613, 55.905) centre (2.4679, 55.4829) ccw
  line L76 (3.175, 54.7758) -> (3.175, 47.2242)
  arc A36 (1.5613, 46.095) -> (3.175, 47.2242) centre (2.4679, 46.5171) ccw
  line L77 (1.5613, 46.095) -> (0, 46.095)
  line L78 (0, 46.095) -> (0, 35.905)
  line L79 (0, 35.905) -> (1.5613, 35.905)
  arc A37 (3.175, 34.7758) -> (1.5613, 35.905) centre (2.4679, 35.4829) ccw
  line L80 (3.175, 34.7758) -> (3.175, 27.2242)
  arc A38 (1.5613, 26.095) -> (3.175, 27.2242) centre (2.4679, 26.5171) ccw
  line L81 (1.5613, 26.095) -> (0, 26.095)
  line L82 (0, 26.095) -> (0, 15.905)
  line L83 (0, 15.905) -> (1.5613, 15.905)
  arc A39 (3.175, 14.7758) -> (1.5613, 15.905) centre (2.4679, 15.4829) ccw
sketch "pHSUpport" plane through (0, 0, 0) normal (0, 0, 1) x (1, 0, 0)
  line L0 (-126.3121, 423.4789) -> (-0.0021, 423.4789)
  line L1 (-0.0021, 423.4789) -> (-0.0021, 307.4298)
  line L2 (-63.1571, 307.4298) -> (-126.3121, 307.4298)
  line L3 (-126.3121, 307.4298) -> (-126.3121, 423.4789)
  circle A0 centre (-95.0428, 331.8598) radius 15
  line L4 (-63.1571, 307.4298) -> (-63.1571, 368.1283)
  line L5 (-63.1571, 368.1283) -> (-0.0021, 368.1283)
  dimension "d1660" = 30
  constraint horizontal L0
  constraint vertical L1
  constraint horizontal L2
  constraint vertical L3
  constraint perpendicular L2 L4
  constraint coincident L1 L5.end
  constraint perpendicular L1 L5
  measures "d1660" diameter of A0
sketch "Sketch1" plane through (0, 0, 0) normal (0, 0, 1) x (1, 0, 0) in component "Peristaltic Pump Support"
  circle A0 centre (53.5964, 47.8456) radius 1.5
  circle A1 centre (22.5964, 47.8456) radius 1.5
  line L0 (55.0964, 58.3456) -> (55.0964, 6.3456) construction
  circle A2 centre (38.0964, 32.3456) radius 15
  line L1 (21.0964, 58.3456) -> (55.0964, 58.3456) construction
  circle A3 centre (38.0964, 56.8456) radius 1.5
  line L2 (55.0964, 6.3456) -> (21.0964, 6.3456) construction
  circle A4 centre (22.5964, 16.8456) radius 1.5
  line L3 (21.0964, 6.3456) -> (21.0964, 58.3456) construction
  circle A5 centre (53.5964, 16.8456) radius 1.5
  circle A6 centre (38.0964, 7.8456) radius 1.5
  point P0 (38.0964, 6.3456)
  point P1 (21.0964, 32.3456)
  point P2 (38.0964, 58.3456)
  dimension "d1669" = 31
  dimension "d1670" = -31
  dimension "d1673" = 0
  dimension "d1674" = 49
  dimension "d1675" = 30
  dimension "d1676" = 15.5
  dimension "d1677" = 34
  dimension "d1678" = 52
  dimension "d1679" = 15.5
  dimension "d1680" = 3
  dimension "d1681" = 3
  constraint horizontal L1
  constraint perpendicular L0 L1
  constraint parallel L1 L2
  constraint parallel L0 L3
  constraint midpoint P1 L3
  constraint horizontal P1 A2.centre
  constraint midpoint P0 L2
  constraint vertical P0 A2.centre
  constraint tangent L2 A6
  constraint midpoint P2 L1
  constraint vertical P2 A3.centre
  measures "d1675" diameter of A2
  measures "d1676" vertical distance of A1.centre A2.centre
  measures "d1677" distance of L0.start L1.start
  measures "d1678" distance of L1.start L2.end
  measures "d1679" horizontal distance of A1.centre A2.centre
  measures "d1680" diameter of A6
  measures "d1681" diameter of A1
equation "fingerWidth = 10 mm"
equation "length = 240 mm"
equation "thickness = 3.175 mm"
equation "height = 60 mm"
equation "d12 = holeWidth"
equation "d13 = thickness"
equation "d14 = thickness"
equation "d15 = thickness"
equation "d21 = lengthCuts"
equation "d23 = -2 * fingerWidth"
equation "toolDiameter = 2 mm"
equation "d34 = toolDiameter"
equation "d36 = boneCenterToHoleSide"
equation "d37 = boneCenterToHoleBottom"
equation "d38 = boneCenterToHoleSide"
equation "boneCenterToHoleBottom = toolDiameter / 2 / sqrt(2) - 0 * kerf" comment "Best: 2.001 -2*kerf, 0.1;;;Best: 2.001 no kerf and 0.1   OLD+6 kerf at 2.001 Diam and .1 mm"
equation "tempLengthPieces = ceil(( ( floor(( length - 2 * thickness ) / fingerWidth) - 2 ) - ( ( floor(( length - 2 * thickness ) / fingerWidth) - 2 ) % 2 - 1 ) ))"
equation "lengthCuts = ceil(tempLengthPieces / 2)"
equation "shoulderToothLength = ( length - fingerWidth * tempLengthPieces ) / 2 - kerf"
equation "depth = 182 mm"
equation "tempDepthPieces = ceil(( ( floor(( depth - 2 * thickness ) / fingerWidth) - 2 ) - ( ( floor(( depth - 2 * thickness ) / fingerWidth) - 2 ) % 2 - 1 ) ))"